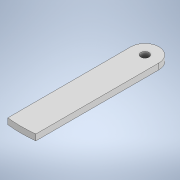
# Autodesk Inventor part: Minute hand test 2
Saved by Autodesk Inventor 2021 (Build 250183000, 183)
## iProperties
Created: 2021-03-29
Part Number: Minute hand test 2
Material: Generic
Document SubType Name: Modeling
Designer: allen
Density: 1 g/cm^3
Appearance: Default
Author: allen
Autodesk Inventor part; units mm, degrees
ref_plane "YZ Plane" through (0, 0, 0) normal (1, 0, 0) x (0, 1, 0)
ref_plane "XZ Plane" through (0, 0, 0) normal (0, 1, 0) x (-1, 0, 0)
ref_plane "XY Plane" through (0, 0, 0) normal (0, 0, 1) x (1, 0, 0)
sketch "Sketch1" plane through (0, 0, 0) normal (0, 1, 0) x (-1, 0, 0)
  circle A0 centre (0, 0) radius 41.5415
  circle A1 centre (0, 0) radius 4.699
  line L0 (4.699, 0) -> (4.699, 41.2749)
  line L1 (-4.699, 0) -> (-4.699, 41.2749)
  dimension "d0" = 83.083
  dimension "d1" = 9.398
  constraints: 4 end point, 4 point on circle, 2 centre point, 2 coincident, 2 tangent, 2 vertical
  measures "d0" diameter of A0
  measures "d1" diameter of A1
extrude "Extrusion1" add sketch "Sketch1" along normal blind 2 contours L0 A1 L1 A0 | A1 picked at (-0.1888, 29.2295)
sketch "Sketch2" plane through (0, 2, 0) normal (0, 1, 0) x (1, 0, 0)
  circle A0 centre (0, 0) radius 1.375
  dimension "d4" = 2.75
  constraints: 1 centre point, 1 coincident
  measures "d4" diameter of A0
extrude "Extrusion2" cut sketch "Sketch2" against normal through all
sketch "Sketch3" plane through (0, 2, 0) normal (0, 1, 0) x (1, 0, 0)
  circle A0 centre (0, 0) radius 1.375 projected
  circle A1 centre (0, 0) radius 4.699
  circle A2 centre (0, 0) radius 1.375 projected
  arc A3 (4.699, 0) -> (-4.699, 0) centre (0, 0) ccw projected
  line L0 (-4.699, 0) -> (-4.699, -41.2749) projected
  arc A4 (-4.699, -41.2749) -> (4.699, -41.2749) centre (0, 0) ccw projected
  line L1 (4.699, -41.2749) -> (4.699, 0) projected
  arc A5 (4.699, 0) -> (-4.699, 0) centre (0, 0) ccw projected
  point P0 (-4.699, 0)
  constraints: 1 centre point, 1 coincident, 1 concentric
body "Solid1"
